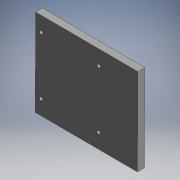
# Autodesk Inventor part: Part14
Saved by Autodesk Inventor 2016 (Build 200138000, 138)
## iProperties
Created: 2018-01-18
Part Number: Part14
Material: Generic
Document SubType Name: Modeling
Designer: student
Density: 1 g/cm^3
Appearance: Default
Author: student
Autodesk Inventor part; units mm, degrees
ref_plane "YZ Plane" through (0, 0, 0) normal (1, 0, 0) x (0, 1, 0)
ref_plane "XZ Plane" through (0, 0, 0) normal (0, 1, 0) x (-1, 0, 0)
ref_plane "XY Plane" through (0, 0, 0) normal (0, 0, 1) x (1, 0, 0)
sketch "Sketch1" plane through (0, 0, 0) normal (0, 0, 1) x (1, 0, 0)
  circle A0 centre (0.2751, 52.8541) radius 1.4214
  circle A1 centre (53.1386, 52.6394) radius 1.4214
  circle A2 centre (52.924, -0.224) radius 1.4214
  circle A3 centre (0.0605, -0.0094) radius 1.4214
  circle A4 centre (0.2751, 52.8541) radius 1.4214
  circle A5 centre (0.0605, -0.0094) radius 1.4214
  circle A6 centre (52.924, -0.224) radius 1.4214
  circle A7 centre (53.1386, 52.6394) radius 1.4214
  line L0 (-5.2574, -13.5336) -> (88.7226, -13.9152)
  line L1 (88.7226, -13.9152) -> (89.0474, 66.0848)
  line L2 (89.0474, 66.0848) -> (-4.9326, 66.4664)
  line L3 (-4.9326, 66.4664) -> (-5.2574, -13.5336)
  line L4 (-5.2574, -13.5336) -> (2.992, -13.5445) construction
  circle A8 centre (26.5572, 26.3424) radius 11 construction
  circle A9 centre (41.9941, 10.7796) radius 1.5 construction
  circle A10 centre (10.9944, 10.9055) radius 1.5 construction
  circle A11 centre (11.1202, 41.9052) radius 1.5 construction
  circle A12 centre (42.12, 41.7793) radius 1.5 construction
  circle A13 centre (0.2148, 52.8996) radius 1.4224 construction
  circle A14 centre (0, 0) radius 1.4224 construction
  circle A15 centre (52.8996, -0.2148) radius 1.4224 construction
  circle A16 centre (53.1143, 52.6848) radius 1.4224 construction
  line L5 (-5.3215, -5.2784) -> (58.178, -5.5363) construction
  line L6 (58.178, -5.5363) -> (58.4358, 57.9632) construction
  line L7 (58.4358, 57.9632) -> (-5.0637, 58.221) construction
  line L8 (-5.0637, 58.221) -> (-5.3215, -5.2784) construction
  point P0 (0.0605, -0.0094)
  point P1 (88.9156, 66.1637)
  dimension "d7" = 80
  dimension "d8" = 93.98
  constraints: 10 end point, 8 centre point, 4 parallel
  measures "d7" vertical distance of L0.end L1.end
  measures "d8" horizontal distance of L1.end L2.end
extrude "Extrusion1" add sketch "Sketch1" along normal blind 6.35
body "Solid1"
